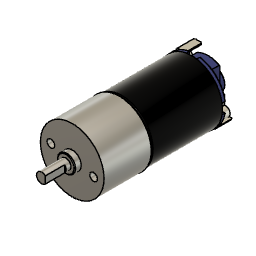
Main Bot v20 (Autodesk Fusion 360 archive; units mm, degrees)
design "CHR-GM25-370 motor"
Autodesk Fusion 360 part; units mm, degrees
sketch "Sketch2" plane through (0, 0, 0) normal (0, 0, 1) x (1, 0, 0)
  circle A0 centre (0, 0) radius 12.45
  circle A1 centre (0, 0) radius 12.15
  circle A2 centre (0, 0) radius 3.5
  circle A3 centre (0, 0) radius 2
  line L0 (-1.3775, 1.45) -> (1.3775, 1.45)
  circle A4 centre (1.476, 8.3709) radius 1.5
  circle A5 centre (-1.476, -8.3709) radius 1.5
  line L1 (1.476, 8.3709) -> (-1.476, -8.3709) construction
  dimension "d6" = 24.9
  dimension "d7" = 24.3
  dimension "d8" = 7
  dimension "d9" = 4
  dimension "d10" = 3.45
  dimension "d17" = 3
  dimension "d18" = 3
  dimension "d19" = 14
  dimension "d1" = 100
  constraint coincident A0.centre A1.centre
  constraint concentric A0 A2
  constraint coincident A3 L0.start
  constraint coincident A3 L0.end
  constraint horizontal L0
  constraint coincident A4.centre L1.start
  constraint coincident A5.centre L1.end
  constraint midpoint A0.centre L1
  measures "d6" diameter of A0
  measures "d7" diameter of A1
  measures "d8" diameter of A2
  measures "d9" diameter of A3
  measures "d17" diameter of A4
  measures "d18" diameter of A5
  measures "d19" distance of A4 A5
  measures "d1" angle of L0 L1
extrude "Extrude1" add sketch "Sketch2" along normal blind 2.5 contours A2 picked at (-2.9183, 0.6668) makes body 1
extrude "Extrude2" add sketch "Sketch2" along normal blind 12 separate body contours A3 L0 picked at (-0.3727, 0.3028) makes body 2
extrude "Extrude3" add sketch "Sketch2" along normal blind 4.4 contours A3 L0 picked at (-0.3882, 1.5086) bodies 2
extrude "Extrude4" add sketch "Sketch2" against normal blind 19 contours A0 | A1 | A2 | A4 | A5 picked at (-12.074, -2.4454) picked at (5.2153, 5.4473) picked at (-2.9183, 0.6668) picked at (1.3425, 8.711) picked at (-1.2581, -8.0419) bodies 1
extrude "Extrude5" cut sketch "Sketch2" against normal blind 4.7 contours A4 | A5 picked at (1.3425, 8.711) picked at (-1.2581, -8.0419) bodies 1
extrude "Extrude6" add sketch "Sketch2" against normal blind 27.7 from surface at -19 separate body contours A1 | A2 | A4 | A5 picked at (5.2153, 5.4473) picked at (-2.9183, 0.6668) picked at (1.3425, 8.711) picked at (-1.2581, -8.0419) makes body 3
fillet "Fillet1" radius 0.5 1 edges at (-11.6075, 4.5021, -19) on bodies 1 3
fillet "Fillet1" radius 0.5 1 edges at (-11.3278, -4.3936, -19) on bodies 1 3
chamfer "Chamfer1" distance 0.3 angle 45 1 edges at (-3.2631, -1.2657, 2.5) on bodies 1
sketch "Sketch3" plane through (0, 0, -46.7) normal (0, 0, -1) x (-1, 0, 0)
  circle A0 centre (0, 0) radius 12.15
  line L0 (0, 12.15) -> (0, -12.15) construction
  line L1 (-12.15, 0) -> (12.15, 0) construction
  line L2 (-2, -11.9843) -> (-2, -4.35)
  line L3 (-9.65, 0) -> (-9.65, -2)
  line L4 (-9.65, -2) -> (-11.9843, -2)
  arc A1 (-8.9, 0) -> (-7.7645, -4.35) centre (0, 0) ccw
  line L5 (-7.7645, -4.35) -> (0, -4.35)
  line L6 (2, -11.9843) -> (2, -4.35)
  line L7 (7.7645, -4.35) -> (0, -4.35)
  arc A2 (7.7645, -4.35) -> (8.9, 0) centre (0, 0) ccw
  line L8 (9.65, 0) -> (9.65, -2)
  line L9 (9.65, -2) -> (11.9843, -2)
  line L10 (2, 11.9843) -> (2, 4.35)
  line L11 (7.7645, 4.35) -> (0, 4.35)
  line L12 (-7.7645, 4.35) -> (0, 4.35)
  line L13 (-2, 11.9843) -> (-2, 4.35)
  arc A3 (-7.7645, 4.35) -> (-8.9, 0) centre (0, 0) ccw
  line L14 (-9.65, 2) -> (-11.9843, 2)
  line L15 (-9.65, 0) -> (-9.65, 2)
  arc A4 (8.9, 0) -> (7.7645, 4.35) centre (0, 0) ccw
  line L16 (9.65, 0) -> (9.65, 2)
  line L17 (9.65, 2) -> (11.9843, 2)
  arc A5 (-11.9843, -2) -> (-2, -11.9843) centre (0, 0) ccw
  arc A6 (2, -11.9843) -> (11.9843, -2) centre (0, 0) ccw
  arc A7 (11.9843, 2) -> (2, 11.9843) centre (0, 0) ccw
  arc A8 (-2, 11.9843) -> (-11.9843, 2) centre (0, 0) ccw
  circle A9 centre (0, 0) radius 4.35
  circle A10 centre (0, 0) radius 1.5
  line L18 (-2, -9.15) -> (0, -9.15)
  line L19 (2, -9.15) -> (0, -9.15)
  line L20 (2, 9.15) -> (0, 9.15)
  line L21 (-2, 9.15) -> (0, 9.15)
  circle A11 centre (6, -7.3) radius 1.85
  line L22 (0, -7.35) -> (-0.6, -7.35)
  line L23 (-0.6, -7.35) -> (-0.6, -5.35)
  line L24 (-0.6, -5.35) -> (0, -5.35)
  line L25 (0.6, -7.35) -> (0.6, -5.35)
  line L26 (0.6, -5.35) -> (0, -5.35)
  line L27 (0, -7.35) -> (0.6, -7.35)
  line L28 (0.6, 7.35) -> (0.6, 5.35)
  line L29 (0, 7.35) -> (0.6, 7.35)
  line L30 (0, 7.35) -> (-0.6, 7.35)
  line L31 (-0.6, 7.35) -> (-0.6, 5.35)
  line L32 (-0.6, 5.35) -> (0, 5.35)
  line L33 (0.6, 5.35) -> (0, 5.35)
  line L34 (7.7645, -4.35) -> (10.0721, -4.35)
  line L35 (10.0721, -4.35) -> (10.0721, -7.35)
  line L36 (10.0721, -7.35) -> (6.5, -9.15)
  line L37 (6.5, -9.15) -> (2, -9.15)
  line L38 (9.5721, -4.35) -> (9.5721, -7.602)
  line L39 (-6.5, 9.15) -> (-2, 9.15)
  circle A12 centre (-6, 7.3) radius 1.85
  line L40 (-10.0721, 7.35) -> (-6.5, 9.15)
  line L41 (-9.5721, 4.35) -> (-9.5721, 7.602)
  line L42 (-10.0721, 4.35) -> (-10.0721, 7.35)
  line L43 (-7.7645, 4.35) -> (-10.0721, 4.35)
  dimension "d33" = 2
  dimension "d35" = 7.8
  dimension "d36" = 2.5
  dimension "d37" = 2
  dimension "d38" = 8.9
  dimension "d39" = 4.35
  dimension "d40" = 3
  dimension "d51" = 3
  dimension "d54" = 3.7
  dimension "d61" = 0.6
  dimension "d62" = 2
  dimension "d63" = 1
  dimension "d67" = 6
  dimension "d68" = 3
  dimension "d70" = 8.5
  dimension "d71" = 4
  dimension "d72" = 0.5
  dimension "d74" = 360
  constraint coincident A0 L0.start
  constraint coincident A0 L0.end
  constraint vertical L0
  constraint midpoint A0.centre L0
  constraint coincident A0 L1.start
  constraint coincident A0 L1.end
  constraint horizontal L1
  constraint midpoint L0 L1
  constraint coincident A0 L2.start
  constraint vertical L2
  constraint coincident L0 L5.end
  constraint coincident L1 L3.start
  constraint coincident A0 L4.end
  constraint horizontal L4
  constraint vertical L3
  constraint coincident L1 A1.start
  constraint coincident A0.centre A1.centre
  constraint horizontal L5
  constraint coincident L2.end L5
  constraint symmetric L0 L2.start L6.start
  constraint symmetric L0 L2.end L6.end
  constraint symmetric L0 L5.end L7.end
  constraint symmetric L0 L3.start L8.start
  constraint symmetric L0 L3.end L8.end
  constraint symmetric L0 L4.end L9.end
  constraint symmetric L0 A1.start A2.end
  constraint symmetric L0 A1.end L7.start
  constraint symmetric L0 A1 A2
  constraint symmetric L1 L2.start L13.start
  constraint symmetric L1 L2.end L13.end
  constraint symmetric L1 L5.end L11.end
  constraint symmetric L1 L3.start L15.start
  constraint symmetric L1 L3.end L14.start
  constraint symmetric L1 L4.end L14.end
  constraint symmetric L1 A1.start A3.end
  constraint symmetric L1 A1.end L12.start
  constraint symmetric L1 A1 A3
  constraint symmetric L1 L6.start L10.start
  constraint symmetric L1 L6.end L10.end
  constraint symmetric L1 L7.start L11.start
  constraint symmetric L1 A2.end A4.start
  constraint symmetric L1 A2 A4
  constraint symmetric L1 L8.start L16.start
  constraint symmetric L1 L8.end L16.end
  constraint symmetric L1 L9.end L17.end
  constraint symmetric L0 A5 A6
  constraint symmetric L1 A5 A8
  constraint symmetric L1 A6 A7
  constraint concentric A5 A9
  constraint coincident L5.end A9
  constraint concentric A3 A10
  constraint coincident L2 L18.start
  constraint coincident L0 L18.end
  constraint horizontal L18
  constraint symmetric L0 L18.start L19.start
  constraint symmetric L0 L18.end L19.end
  constraint symmetric L1 L18.start L21.start
  constraint symmetric L1 L18.end L20.end
  constraint symmetric L1 L19.start L20.start
  constraint coincident L0 L22.start
  constraint coincident L0 L24.end
  constraint horizontal L22
  constraint vertical L23
  constraint horizontal L24
  constraint symmetric L0 L22.start L27.start
  constraint symmetric L0 L22.end L25.start
  constraint symmetric L0 L23.end L25.end
  constraint symmetric L0 L24.end L26.end
  constraint symmetric L1 L22.start L29.start
  constraint symmetric L1 L22.end L30.end
  constraint symmetric L1 L23.end L31.end
  constraint symmetric L1 L24.end L32.end
  constraint symmetric L1 L25.start L28.start
  constraint symmetric L1 L25.end L28.end
  constraint horizontal L34
  constraint horizontal L37
  constraint vertical L35
  constraint tangent A11 L37
  constraint coincident L34 L38.start
  constraint coincident L36 L38.end
  constraint vertical L38
  measures "d33" distance of L2.end L5.end
  measures "d35" distance of L0.end L5.end
  measures "d36" distance of L1.start L3.start
  measures "d37" distance of L3.start L3.end
  measures "d38" radius of A1
  measures "d39" distance of L1 L5
  measures "d40" diameter of A10
  measures "d51" distance of L0.end L18.end
  measures "d54" diameter of A11
  measures "d61" horizontal distance of L22.start L22.end
  measures "d62" distance of L22.end L23.end
  measures "d63" distance of L5 L24
  measures "d67" distance of L0 A11.centre
  measures "d68" distance of L34.end L35.end
  measures "d70" distance of L18.start L36.end
  measures "d71" distance of L35.end L36.end
  measures "d72" distance of L35 L38
extrude "Extrude7" add sketch "Sketch3" along normal blind 1.5 separate body contours A0 A2 L8 L9 L10 L11 A4 L16 L17 A6 A7 L34 L35 | A0 A6 L34 L35 L38 | A0 L13 A8 L39 L40 | A11 | A0 L6 L7 A6 L34 L36 L37 L38 | A12 | A0 L12 L13 A8 L39 L40 L41 L43 | L7 A2 L11 A4 A9 | A0 L6 A6 L36 L37 | A0 A8 L41 L42 L43 | A1 L5 L12 A3 A9 | A9 | A0 L2 L3 L4 A1 L5 A3 L14 L15 A5 A8 L42 L43 picked at (5.47, 7.8905) picked at (9.9054, -5.1651) picked at (-4.4419, 9.7402) picked at (6.6817, -7.942) picked at (2.7285, -6.813) picked at (-6.5504, 7.8488) picked at (-2.7233, 6.8428) picked at (4.2044, 3.9958) picked at (4.4419, -9.7402) picked at (-9.9054, 5.1651) picked at (-4.2411, 3.9629) picked at (-2.8025, 1.9107) picked at (-5.47, -7.8905) makes body 4
extrude "Extrude8" add sketch "Sketch3" along normal blind 5.3 from surface at 1.5 contours L7 A2 L11 A4 A9 | A1 L5 L12 A3 A9 | A9 picked at (4.2044, 3.9958) picked at (-4.2411, 3.9629) picked at (-2.8025, 1.9107) bodies 4
extrude "Extrude9" add sketch "Sketch3" along normal blind 2.2 from surface at 6.8 contours A9 picked at (-2.8025, 1.9107) bodies 4
extrude "Extrude10" add 1 faces at (0.637, 0.1965, 0) along direction (0, 0, -1) up to surface (54.7 mm away) on bodies 2 bodies 2
extrude "Extrude11" add sketch "Sketch3" along normal blind 3.8 separate body contours L10 L11 L12 L13 L20 L21 | L2 L5 L6 L7 L18 L19 | L22 L23 L24 L25 L26 L27 | L28 L29 L30 L31 L32 L33 picked at (1.5333, 6.95) picked at (1.5333, -6.95) picked at (-0.2, -6.6833) picked at (-0.2, 6.6833) makes body 5 at (-0.6667, -7.55, -46.7) makes body 6 at (-0.6667, 7.55, -46.7)
extrude "Extrude13" add sketch "Sketch3" along normal blind 1.3 from surface at 3.8 contours L22 L23 L24 L25 L26 L27 | L28 L29 L30 L31 L32 L33 picked at (-0.2, -6.6833) picked at (-0.2, 6.6833) bodies 5 6
extrude "Extrude12" add sketch "Sketch3" along normal blind 0.5 from surface at 1.5 contours A0 A6 L35 L36 | A0 A6 L34 L35 L38 | A12 | A11 | L6 L7 L34 L36 L37 L38 | A0 A8 L41 L42 L43 | A0 A8 L40 L42 | L12 L13 L39 L40 L41 L43 picked at (9.8906, -7.237) picked at (9.9054, -5.1651) picked at (-5.3785, 7.6945) picked at (4.8614, -6.7744) picked at (2.7181, -6.8915) picked at (-9.9054, 5.1651) picked at (-9.8906, 7.237) picked at (-2.7234, 6.8422) bodies 5 6
extrude "Extrude14" add sketch "Sketch3" along normal blind 4 from surface at 2 contours A11 | A12 picked at (6.6817, -7.942) picked at (-6.5504, 7.8488) bodies 5 6
extrude "Extrude15" add sketch "Sketch3" along normal blind 6.5 from surface at 2 contours A0 A6 L35 L36 L38 | A0 A6 L34 L35 L38 | A0 A8 L41 L42 L43 | A0 A8 L40 L41 L42 picked at (9.909, -7.212) picked at (9.9054, -5.1651) picked at (-9.9054, 5.1651) picked at (-9.909, 7.212) bodies 5 6
fillet "Fillet2" radius 0.3 14 edges at (8.5913, -8.5913, -48.2) (10.8171, -2, -48.2) (9.65, 0, -48.2) (10.8171, 2, -48.2) (8.5913, 8.5913, -48.2) (2, 8.1671, -48.2) (-2, 8.1671, -48.2) (2, -8.1671, -48.2) (-2, -8.1671, -48.2) (-8.5913, -8.5913, -48.2) (-10.8171, -2, -48.2) (-9.65, 0, -48.2) (-10.8171, 2, -48.2) (-8.5913, 8.5913, -48.2) on bodies 4
fillet "Fillet2" radius 0.3 2 edges at (8.9, 0, -53.5) (-8.9, 0, -53.5) on bodies 4
fillet "Fillet2" radius 0.3 1 edges at (4.0556, -1.573, -55.7) on bodies 4
fillet "Fillet3" radius 0.5 2 edges at (0, -7.35, -51.8) (0, 7.35, -51.8) on bodies 5 6
fillet "Fillet3" radius 0.3 4 edges at (2, -6.75, -50.5) (-2, -6.75, -50.5) (2, 6.75, -50.5) (-2, 6.75, -50.5) on bodies 5 6
fillet "Fillet3" radius 0.3 3 edges at (-10.0721, -5.85, -48.2) (-9.8221, -7.476, -55.2) (-9.8221, -4.35, -55.2) on bodies 5 6
fillet "Fillet3" radius 0.3 3 edges at (10.0721, 5.85, -48.2) (9.8221, 7.476, -55.2) (9.8221, 4.35, -55.2) on bodies 5 6
move_body "Move1" bodies 6 4 2 1 3 5 to x (0, -1, 0) y (1, 0, 0) z (0, 0, 1) at (0, 0, 0)
sketch "Shape" plane through (0, 0, 0) normal (0, 1, 0) x (1, 0, 0)
  line L0 (3.5, 0) -> (12.45, 0) construction
  line L1 (-12.45, 0) -> (-3.5, 0) construction
  line L2 (3.2, -2.5) -> (3.5, -2.2) construction
  line L3 (-3.2, -2.5) -> (-3.5, -2.2) construction
  line L4 (-3.5, 0) -> (-3.5, -2.2) construction
  line L5 (3.5, 0) -> (3.5, -2.2) construction
  arc A0 (-11.95, 19) -> (-12.45, 18.5) centre (-11.95, 18.5) ccw construction
  arc A1 (12.45, 18.5) -> (11.95, 19) centre (11.95, 18.5) ccw construction
  line L6 (12.45, 0) -> (12.45, 18.5) construction
  line L7 (-12.45, 0) -> (-12.45, 18.5) construction
  arc A2 (11.65, 19) -> (12.15, 19.5) centre (11.65, 19.5) ccw construction
  arc A3 (-12.15, 19.5) -> (-11.65, 19) centre (-11.65, 19.5) ccw construction
  line L8 (12.15, 19.5) -> (12.15, 46.7) construction
  line L9 (-12.15, 19.5) -> (-12.15, 46.7) construction
  ellipse E0 centre (7.266, 54.9) end of major axis (7.602, 54.9) minor radius 0.3 (7.602, 54.9) -> (7.266, 55.2) ccw
  line L10 (7.602, 52.7) -> (7.602, 54.9) construction
  line L11 (9.15, 52.7) -> (7.602, 52.7) construction
  line L12 (9.15, 48.7) -> (9.15, 52.7) construction
  arc A4 (-4.05, 55.7) -> (-4.35, 55.4) centre (-4.05, 55.4) ccw construction
  arc A5 (4.35, 55.4) -> (4.05, 55.7) centre (4.05, 55.4) ccw construction
  line L13 (4.35, 53.5) -> (4.35, 55.4) construction
  line L14 (-4.35, 53.5) -> (-4.35, 55.4) construction
  line L15 (-7.602, 52.7) -> (-7.602, 54.9) construction
  ellipse E1 centre (-7.266, 54.9) end of major axis (-7.602, 54.9) minor radius 0.3 (-7.266, 55.2) -> (-7.602, 54.9) ccw
  line L16 (-7.602, 52.7) -> (-9.15, 52.7) construction
  line L17 (-9.15, 50.5) -> (-9.15, 52.7) construction
  line L18 (3.5181, 55.5373) -> (0, 0) construction
  line L19 (3.5181, 55.5373) -> (9.15, 55.5373)
  line L20 (9.15, 55.5373) -> (9.15, 48.5975)
  line L21 (9.15, 48.5975) -> (-12.45, 48.5975)
  line L22 (-12.45, 48.5975) -> (-12.45, 0)
  line L23 (-12.45, 0) -> (0, 0)
  line L24 (12.3505, -1.571) -> (0, 0)
  line L25 (18.4829, 46.638) -> (12.3505, -1.571)
  line L26 (3.5181, 55.5373) -> (-2.0687, 56.248)
  line L27 (-2.0687, 56.248) -> (-2.9444, 49.3636)
  line L28 (-2.9444, 49.3636) -> (18.4829, 46.638)
  line L29 (3.2, -2.5) -> (-3.2, -2.5)
  line L30 (-11.95, 19) -> (11.95, 19)
  line L31 (11.65, 19) -> (-11.65, 19)
  line L32 (12.15, 46.7) -> (-12.15, 46.7)
  arc A6 (4.65, 55.2) -> (4.35, 54.9) centre (4.65, 54.9) ccw
  line L33 (4.35, 48.5) -> (4.35, 54.9)
  line L34 (4.35, 48.2) -> (4.35, 48.5)
  line L35 (4.35, 46.7) -> (4.35, 48.2)
  line L36 (7.0141, 55.2) -> (4.65, 55.2)
  line L37 (7.0141, 55.2) -> (7.266, 55.2)
  line L38 (9.15, 48.2) -> (9.15, 48.7)
  line L39 (9.15, 46.7) -> (9.15, 48.2)
  line L40 (9.15, 46.7) -> (4.35, 46.7)
  line L41 (0, 55.7) -> (4.05, 55.7)
  line L42 (-4.05, 55.7) -> (0, 55.7)
  line L43 (-4.35, 53.2) -> (-4.35, 53.5)
  line L44 (-4.35, 48.2) -> (-4.35, 53.2)
  line L45 (4.35, 53.5) -> (4.35, 53.2)
  line L46 (4.35, 48.2) -> (4.35, 53.2)
  spline S0 degree 3 poles (-11.6247, 48.2) (-11.6256, 48.2) (-11.6266, 48.2) (-11.6694, 48.1997) (-11.7115, 48.1935) (-11.7893, 48.1694) (-11.8262, 48.152) (-11.8882, 48.1075) (-11.9149, 48.0817) (-11.9519, 48.0279) (-11.9646, 48.0026) (-11.9804, 47.9508) (-11.9843, 47.9257) (-11.9843, 47.9) knots -0.060627 -0.060627 -0.060627 -0.060627 -0.060246 -0.060246 -0.044216 -0.044216 -0.029361 -0.029361 -0.016715 -0.016715 -0.007714 -0.007714 0 0 0 0
  line L47 (-11.6247, 48.2) -> (-4.35, 48.2)
  line L48 (4.35, 48.2) -> (11.6247, 48.2)
  spline S1 degree 3 poles (11.6247, 48.2) (11.6256, 48.2) (11.6266, 48.2) (11.6694, 48.1997) (11.7115, 48.1935) (11.7893, 48.1694) (11.8262, 48.152) (11.8882, 48.1075) (11.9149, 48.0817) (11.9519, 48.0279) (11.9646, 48.0026) (11.9804, 47.9508) (11.9843, 47.9257) (11.9843, 47.9) knots -0.000386 -0.000386 -0.000386 -0.000386 0 0 0.016218 0.016218 0.031247 0.031247 0.044041 0.044041 0.053148 0.053148 0.060952 0.060952 0.060952 0.060952
  line L49 (-11.9843, 46.7) -> (-11.9843, 47.9)
  line L50 (-2, 46.7) -> (-11.9843, 46.7)
  line L51 (-2, 46.7) -> (2, 46.7)
  line L52 (11.9843, 46.7) -> (11.9843, 47.9)
  line L53 (11.9843, 46.7) -> (2, 46.7)
  arc A7 (-4.35, 54.9) -> (-4.65, 55.2) centre (-4.65, 54.9) ccw
  line L54 (-4.65, 55.2) -> (-7.266, 55.2)
  line L55 (-4.35, 50.5) -> (-4.35, 54.9)
  line L56 (-9.15, 50.2) -> (-9.15, 50.5)
  line L57 (-9.15, 46.7) -> (-9.15, 50.2)
  line L58 (-4.35, 50.5) -> (-4.35, 50.2)
  line L59 (-4.35, 46.7) -> (-4.35, 50.2)
  line L60 (-9.15, 46.7) -> (-4.35, 46.7)
  constraint coincident L18.end L23.end
  constraint horizontal L19
  constraint horizontal L21
  constraint vertical L20
  constraint collinear L12 L20
  constraint horizontal L23
  constraint vertical L22
  constraint coincident L21.end L22.start
  constraint collinear L7 L22
  constraint symmetric L19.start L18 L26.start
  constraint symmetric L18 L19.end L26.end
  constraint symmetric L18 L20.end L27.end
  constraint symmetric L18 L21.end L25.start
  constraint symmetric L18 L1.start L24.start
  constraint symmetric L18 L23.end L24.end
equation "d25 = -46.7 mm + 19 mm"
equation "d38 = ( 17.8 / 2 ) * 1 mm"
named bodies: "Shaft"
